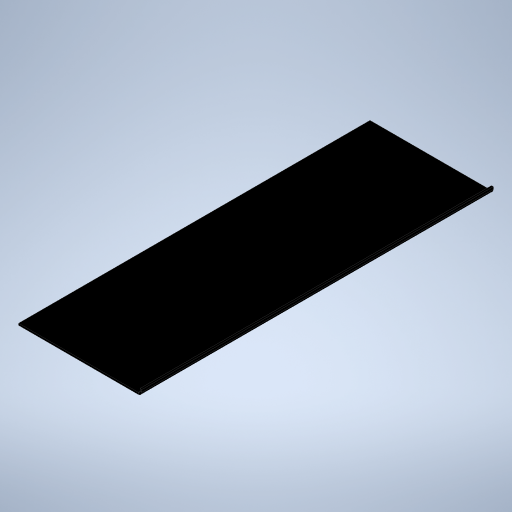
# Autodesk Inventor part: CO-1-01-controlsSeperator
Saved by Autodesk Inventor 2023 (Build 270158000, 158)
## iProperties
Created: 2023-04-06
Part Number: CO-1-01-controlsSeperator
Material: Generic
Document SubType Name: Sheet Metal
Designer: t205b
Density: 1 g/cm^3
Sheet Metal Rule: Default
Appearance: Default
Author: t205b
Autodesk Inventor part; units mm, degrees
ref_plane "YZ Plane" through (0, 0, 0) normal (1, 0, 0) x (0, 1, 0)
ref_plane "XZ Plane" through (0, 0, 0) normal (0, 1, 0) x (-1, 0, 0)
ref_plane "XY Plane" through (0, 0, 0) normal (0, 0, 1) x (1, 0, 0)
sketch "Sketch1" plane through (0, 0, 0) normal (0, 1, 0) x (-1, 0, 0)
  line L0 (97, 285) -> (-97, 285)
  line L1 (-97, 285) -> (-97, -285)
  line L2 (-97, -285) -> (97, -285)
  line L3 (97, -285) -> (97, 285)
  point P0 (0, 0)
  dimension "d0" = 194
  dimension "d1" = 570
  dimension "d2" = 97
  dimension "d3" = 285
  measures "d0" distance between parallel lines of L1 L3
  measures "d1" distance of L2.end L0.start
  measures "d2" distance from line of L3 point (0, 0)
  measures "d3" distance from line of point (0, 0) L2
extrude "Plate1" add sketch "Sketch1" along normal blind 3.048
sketch "Sketch3" plane through (100.048, 6.096, -285) normal (1, 0, 0) x (0, 1, 0)
  line L0 (0, 570) -> (0, 0)
  line L1 (0, 0) -> (3.904, 0)
  line L2 (3.904, 0) -> (3.904, 570)
  line L3 (3.904, 570) -> (0, 570)
  constraints: 6 end point, 1 horizontal, 1 perpendicular, 1 vertical
edge flange "Flange1" height 10 angle 90 thickness 3.048 bend radius 3.048 thickness toward (1, 0, 0) relief tear relief width 3.048 relief depth 1.524 edges at (97, 3.048, 0) wall of the first edge with corners at (100.048, 6.096, 285) (100.048, 6.096, -285) (100.048, 10, -285) (100.048, 10, 285)
bend "Bend1"
corner "Corner1"
equation "\"d4\" = Thickness"
equation "\"d5\" = BendReliefWidth"
equation "\"d6\" = BendReliefDepth"
equation "\"d7\" = MinimumRemnant"
equation "\"d8\" = TransitionRadius"
equation "\"d11\" = BendRadius"
equation "\"d12\" = CornerReliefSize"
equation "\"d13\" = GapSize"
equation "\"d14\" = JacobiRadiusSize"
equation "\"d2\" = 0.5 * d0"
equation "\"d3\" = 0.5 * d1"
equation "\"BendRadius\" = Thickness"
equation "\"BendReliefWidth\" = Thickness"
equation "\"BendReliefDepth\" = 0.5 * Thickness"
equation "\"CornerReliefSize\" = 4 * Thickness"
equation "\"MinimumRemnant\" = 2 * Thickness"
equation "\"TransitionRadius\" = BendRadius"
equation "\"JacobiRadiusSize\" = BendRadius"
equation "\"GapSize\" = Thickness"
equation "\"Thickness\" = 3.048"
body "Solid1"
